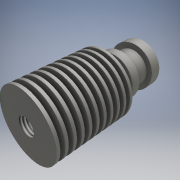
# Autodesk Inventor part: Heatsink
Saved by Autodesk Inventor 2016 (Build 200138000, 138)
## iProperties
Created: 2016-03-26
Part Number: Heatsink
Material: Aluminum 6061
Document SubType Name: Modeling
Designer: Scott
Density: 2.7 g/cm^3
Appearance: Aluminum - Flat
Mass: 19.313 g
Surface Area: 99.7958 cm^2
Volume: 7.15295 cm^3
Author: Scott
Autodesk Inventor part; units mm, degrees
ref_plane "YZ Plane" through (0, 0, 0) normal (1, 0, 0) x (0, 1, 0)
ref_plane "XZ Plane" through (0, 0, 0) normal (0, 1, 0) x (-1, 0, 0)
ref_plane "XY Plane" through (0, 0, 0) normal (0, 0, 1) x (1, 0, 0)
sketch "Sketch1" plane through (0, 0, 0) normal (0, 0, 1) x (1, 0, 0)
  line L0 (0, 0) -> (11.15, 0)
  line L1 (11.15, 0) -> (11.15, 26)
  line L2 (11.15, 26) -> (8, 26)
  line L3 (8, 42.7) -> (0, 42.7)
  line L4 (0, 42.7) -> (0, 0)
  line L5 (8, 39) -> (6, 39)
  line L6 (6, 39) -> (6, 33)
  line L7 (6, 33) -> (8, 33)
  line L8 (8, 26) -> (5, 26)
  line L9 (5, 26) -> (5, 27.5)
  line L10 (5, 27.5) -> (8, 27.5)
  line L11 (8, 28.5) -> (5, 28.5)
  line L12 (5, 28.5) -> (5, 30)
  line L13 (5, 30) -> (8, 30)
  line L14 (8, 39) -> (8, 42.7)
  line L15 (8, 27.5) -> (8, 28.5)
  line L16 (8, 30) -> (8, 33)
  dimension "d7" = 11.15
  dimension "d10" = 8
  dimension "d11" = 42.7
  dimension "d12" = 26
  dimension "d14" = 6
  dimension "d15" = 3.7
  dimension "d16" = 3
  dimension "d17" = 6
  dimension "d18" = 1
  dimension "d19" = 2.5
  dimension "d20" = 5
  constraints: 34 end point, 19 perpendicular, 3 horizontal, 2 collinear, 2 parallel, 2 point on line
  measures "d7" distance between parallel lines of L1 L4
  measures "d10" distance of L3.start L3.end
  measures "d11" distance between parallel lines of L0 L3
  measures "d12" distance of L0.end L1.end
  measures "d14" distance between parallel lines of L4 L6
  measures "d15" distance of L5.start L3.start
  measures "d16" distance of L13.end L7.end
  measures "d17" distance of L5.end L6.end
  measures "d18" distance of L10.end L11.start
  measures "d19" distance between parallel lines of L2 L11
  measures "d20" distance between parallel lines of L4 L12
revolve "Revolution1" add sketch "Sketch1" angle 360 about axis through (0, 42.7, 0) along (0, -1, 0)
sketch "Sketch2" plane through (0, 42.7, 0) normal (0, 1, 0) x (1, 0, 0)
  circle A0 centre (0, 0) radius 8 projected
  circle A1 centre (0, 0) radius 8 projected
hole "Hole1" at (0, 42.7, 0) direction (0, -1, 0) diameter 4.2 end through all
sketch "Sketch3" plane through (0, 42.7, 0) normal (0, 1, 0) x (1, 0, 0)
  circle A0 centre (0, 0) radius 2.1 projected
  circle A1 centre (0, 0) radius 8 projected
hole "Hole2" at (0, 42.7, 0) direction (0, -1, 0) diameter 8 depth 6 tip angle 118
sketch "Sketch4" plane through (0, 0, 0) normal (0, -1, 0) x (1, 0, 0)
  circle A0 centre (0, 0) radius 2.1 projected
  circle A1 centre (0, 0) radius 11.15 projected
hole "Hole3" at (0, 0, 0) direction (0, 1, 0) diameter 5.917 depth 19.1 tip angle 118 thread size "M7x1" class "6H" standard "ISO Metric profile"
sketch "Sketch5" plane through (0, 0, 0) normal (0, 0, 1) x (1, 0, 0)
  line L0 (5, 27.5) -> (5, 26) projected
  line L1 (-11.15, 26) -> (11.15, 26) projected
  line L2 (11.15, 26) -> (11.15, 0) projected
  line L3 (-11.15, 0) -> (11.15, 0) projected
  line L4 (5, 26) -> (6.15, 0)
  line L5 (11.15, 2.5) -> (6.1058, 2.5)
  line L6 (6.1058, 2.5) -> (6.1058, 1)
  line L7 (6.1058, 1) -> (11.15, 1)
  line L8 (11.15, 1) -> (11.15, 2.5)
  line L9 (11.15, 5) -> (5.9952, 5)
  line L10 (5.9952, 5) -> (5.9952, 3.5)
  line L11 (5.9952, 3.5) -> (11.15, 3.5)
  line L12 (11.15, 3.5) -> (11.15, 5)
  line L13 (11.15, 7.5) -> (5.8846, 7.5)
  line L14 (5.8846, 7.5) -> (5.8846, 6)
  line L15 (5.8846, 6) -> (11.15, 6)
  line L16 (11.15, 6) -> (11.15, 7.5)
  line L17 (11.15, 10) -> (5.774, 10)
  line L18 (5.774, 10) -> (5.774, 8.5)
  line L19 (5.774, 8.5) -> (11.15, 8.5)
  line L20 (11.15, 8.5) -> (11.15, 10)
  line L21 (11.15, 12.5) -> (5.6635, 12.5)
  line L22 (5.6635, 12.5) -> (5.6635, 11)
  line L23 (5.6635, 11) -> (11.15, 11)
  line L24 (11.15, 11) -> (11.15, 12.5)
  line L25 (11.15, 15) -> (5.5529, 15)
  line L26 (5.5529, 15) -> (5.5529, 13.5)
  line L27 (5.5529, 13.5) -> (11.15, 13.5)
  line L28 (11.15, 13.5) -> (11.15, 15)
  line L29 (11.15, 17.5) -> (5.4423, 17.5)
  line L30 (5.4423, 17.5) -> (5.4423, 16)
  line L31 (5.4423, 16) -> (11.15, 16)
  line L32 (11.15, 16) -> (11.15, 17.5)
  line L33 (11.15, 20) -> (5.3317, 20)
  line L34 (5.3317, 20) -> (5.3317, 18.5)
  line L35 (5.3317, 18.5) -> (11.15, 18.5)
  line L36 (11.15, 18.5) -> (11.15, 20)
  line L37 (11.15, 22.5) -> (5.2212, 22.5)
  line L38 (5.2212, 22.5) -> (5.2212, 21)
  line L39 (5.2212, 21) -> (11.15, 21)
  line L40 (11.15, 21) -> (11.15, 22.5)
  line L41 (11.15, 25) -> (5.1106, 25)
  line L42 (5.1106, 25) -> (5.1106, 23.5)
  line L43 (5.1106, 23.5) -> (11.15, 23.5)
  line L44 (11.15, 23.5) -> (11.15, 25)
  line L45 (0, -8.54) -> (0, 51.24) projected
  point P0 (0, 0)
  dimension "d42" = 1
  dimension "d43" = 2.5
  dimension "d46" = 5
  dimension "d47" = 1
  dimension "d48" = 2.5
  dimension "d49" = 1
  dimension "d50" = 2.5
  dimension "d51" = 1
  dimension "d52" = 2.5
  dimension "d53" = 1
  dimension "d54" = 2.5
  dimension "d55" = 1
  dimension "d56" = 2.5
  dimension "d57" = 1
  dimension "d58" = 2.5
  dimension "d59" = 1
  dimension "d60" = 2.5
  dimension "d61" = 1
  dimension "d62" = 2.5
  dimension "d63" = 1
  dimension "d64" = 2.5
  constraints: 80 end point, 20 parallel, 10 horizontal, 10 perpendicular, 1 point on line, 24 other
  measures "d42" distance between parallel lines of L3 L7
  measures "d43" distance between parallel lines of L3 L5
  measures "d46" distance of L3.end point (6.15, 0)
  measures "d47" distance between parallel lines of L11 L5
  measures "d48" distance between parallel lines of L9 L5
  measures "d49" distance from line of L15 L9.start
  measures "d50" distance between parallel lines of L13 L9
  measures "d51" distance between parallel lines of L13 L19
  measures "d52" distance between parallel lines of L17 L13
  measures "d53" distance between parallel lines of L17 L23
  measures "d54" distance between parallel lines of L21 L17
  measures "d55" distance between parallel lines of L21 L27
  measures "d56" distance between parallel lines of L25 L21
  measures "d57" distance between parallel lines of L25 L31
  measures "d58" distance between parallel lines of L29 L25
  measures "d59" distance between parallel lines of L29 L35
  measures "d60" distance between parallel lines of L33 L29
  measures "d61" distance between parallel lines of L39 L33
  measures "d62" distance between parallel lines of L37 L33
  measures "d63" distance between parallel lines of L37 L43
  measures "d64" distance between parallel lines of L41 L37
revolve "Revolution2" cut sketch "Sketch5" angle 360 about axis through (0, -10, 0) along (0, 1, 0) contours L42 L41 L2 L43 | L38 L37 L2 L39 | L34 L33 L2 L35 | L6 L5 L2 L7 | L30 L29 L2 L31 | L10 L9 L2 L11 | L26 L25 L2 L27 | L14 L13 L2 L15 | L22 L21 L2 L23 | L18 L17 L2 L19
equation "\"d47\" = d42"
equation "\"d48\" = d43"
equation "\"d49\" = d42"
equation "\"d50\" = d43"
equation "\"d51\" = d42"
equation "\"d52\" = d43"
equation "\"d53\" = d42"
equation "\"d54\" = d43"
equation "\"d55\" = d42"
equation "\"d56\" = d43"
equation "\"d57\" = d42"
equation "\"d58\" = d43"
equation "\"d59\" = d42"
equation "\"d60\" = d43"
equation "\"d61\" = d42"
equation "\"d62\" = d43"
equation "\"d63\" = d42"
equation "\"d64\" = d43"
body "Solid1"
